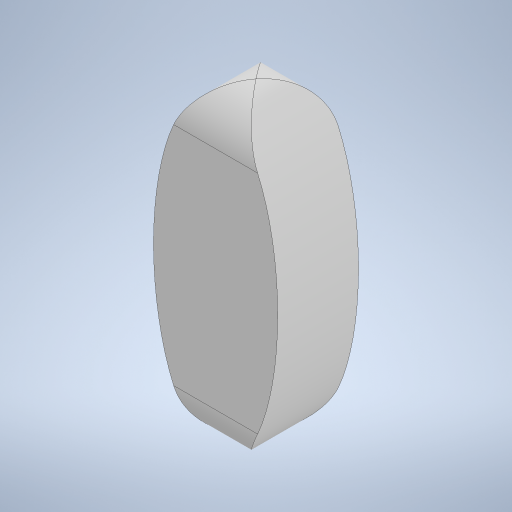
# Autodesk Inventor part: bloqueadorXD
Saved by Autodesk Inventor 2024.4 (Build 284460000, 460)
## iProperties
Created: 2026-06-02
Part Number: bloqueadorXD
Material: Generic
Document SubType Name: Modeling
Designer: Apleppli
Density: 1 g/cm^3
Appearance: Default
Author: Apleppli
Autodesk Inventor part; units mm, degrees
ref_plane "YZ Plane" through (0, 0, 0) normal (1, 0, 0) x (0, 1, 0)
ref_plane "XZ Plane" through (0, 0, 0) normal (0, 1, 0) x (-1, 0, 0)
ref_plane "XY Plane" through (0, 0, 0) normal (0, 0, 1) x (1, 0, 0)
sketch "Sketch1" plane through (0, 0, 0) normal (0, 0, 1) x (1, 0, 0)
  line L0 (3.25, -4.55) -> (-3.25, -4.55)
  line L1 (-3.25, -4.55) -> (-3.25, 4.55)
  line L2 (-3.25, 4.55) -> (3.25, 4.55)
  line L3 (3.25, 4.55) -> (3.25, -4.55)
  line L4 (3.25, -4.55) -> (-3.25, 4.55) construction
  line L5 (-3.25, -4.55) -> (3.25, 4.55) construction
  line L6 (0, 4.55) -> (0, -4.55)
  line L7 (0, 4.55) -> (0, 12.35)
  line L8 (0, -4.55) -> (0, -7.8)
  ellipse E0 centre (0, 0) end of major axis (0, 12.35) minor radius 5
  dimension "d4" = 5
  dimension "d7" = 12.35
  dimension "diametro" = 6.5
  dimension "altura" = 9.1
  dimension "d2" = 3.25
  constraints: 18 end point, 4 midpoint, 3 coincident, 2 parallel, 2 vertical, 1 horizontal, 1 perpendicular, 1 point on line, 1 vertical alignment, 2 other
  measures "diametro" distance of L1.end L2.end
  measures "altura" distance of L0.end L1.end
  measures "d2" distance between parallel lines of L6 L1
extrude "Extrusion1" add sketch "Sketch1" along normal mid plane 6.5 contours L0 L6 L2 L3 | L0 L1 L2 L6 | E0
sketch "Sketch2" plane through (0, 0, 0) normal (1, 0, 0) x (0, 1, 0)
  line L0 (-12.35, -3.25) -> (12.35, -3.25) projected
  line L1 (12.35, 3.25) -> (-12.35, 3.25) projected
  line L2 (-9.1, -3.25) -> (9.1, -3.25)
  line L3 (9.1, -3.25) -> (9.1, 3.25)
  line L4 (9.1, 3.25) -> (-9.1, 3.25)
  line L5 (-9.1, 3.25) -> (-9.1, -3.25)
  line L6 (-9.1, -3.25) -> (9.1, 3.25) construction
  line L7 (9.1, -3.25) -> (-9.1, 3.25) construction
  line L8 (0, 0) -> (9.1, 0)
  circle A0 centre (9.1, 0) radius 3.25
  circle A1 centre (-9.1, 0) radius 3.25
  line L9 (9.1, 0) -> (12.35, 0)
  line L10 (-9.1, 0) -> (-12.35, 0)
  line L11 (-12.35, 3.25) -> (-12.35, -3.25)
  line L12 (12.35, 3.25) -> (12.35, -3.25)
  dimension "d8" = 18.2
  constraints: 22 end point, 4 midpoint, 4 point on circle, 2 centre point, 2 horizontal, 2 parallel, 2 perpendicular, 2 point on line, 1 coincident, 1 vertical
  measures "d8" distance of L4.end L3.end
extrude "Extrusion2" cut sketch "Sketch2" along normal mid plane 60 contours L11 A1 L0 | L11 L1 A1 | A0 L12 L0 | A0 L1 L12
equation "\"d7\" = altura + 0.5 * diametro"
equation "\"d5\" = diametro"
equation "\"d8\" = 2 * altura"
body "Solid2"
